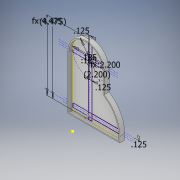
# Autodesk Inventor part: housing
Saved by Autodesk Inventor 2017 (Build 210142000, 142)
## iProperties
Created: 2016-11-23
Part Number: housing
Material: Generic
Document SubType Name: Modeling
Designer: cody
Density: 1 g/cm^3
Appearance: Default
Author: cody
Autodesk Inventor part; units mm, degrees
ref_plane "YZ Plane" through (0, 0, 0) normal (1, 0, 0) x (0, 1, 0)
ref_plane "XZ Plane" through (0, 0, 0) normal (0, 1, 0) x (-1, 0, 0)
ref_plane "XY Plane" through (0, 0, 0) normal (0, 0, 1) x (1, 0, 0)
sketch "Outline" plane through (0, 0, 0) normal (0, 0, 1) x (1, 0, 0)
  line L0 (0, 37.1721) -> (55.88, 37.1721) construction
  line L1 (55.88, 37.1721) -> (55.88, 115.2771) construction
  line L2 (55.88, 115.2771) -> (0, 115.2771) construction
  line L3 (0, 115.2771) -> (0, 37.1721) construction
  circle A0 centre (27.94, 115.2771) radius 26.67 construction
  circle A1 centre (27.94, 37.1721) radius 52.07 construction
  circle A2 centre (27.94, 115.2771) radius 27.94 construction
  circle A3 centre (27.94, 37.1721) radius 53.34 construction
  arc A4 (55.88, 115.2771) -> (0, 115.2771) centre (27.94, 115.2771) ccw
  line L4 (55.88, 115.2771) -> (55.88, 82.609)
  arc A5 (81.28, 37.1721) -> (55.88, 82.609) centre (27.94, 37.1721) ccw
  line L5 (142.2611, 29.5521) -> (-127.7704, 29.5521) construction
  line L6 (81.28, 37.1721) -> (81.28, 29.5521)
  line L7 (0, 29.5521) -> (81.28, 29.5521)
  line L8 (0, 115.2771) -> (0, 29.5521)
  dimension "d20" = 78.105
  dimension "d23" = 104.14
  dimension "d25" = 53.34
  dimension "d27" = 1.27
  dimension "d28" = 55.88
  dimension "d29" = 55.88
  dimension "d30" = 1.27
  dimension "d31" = 7.62
  constraints: 18 end point, 5 centre point, 4 point on circle, 3 horizontal, 3 point on line, 3 vertical, 2 midpoint, 2 parallel, 2 perpendicular, 1 coincident, 1 collinear, 1 tangent, 3 other
  measures "d20" distance of L2.end L0.start
  measures "d23" diameter of A1
  measures "d25" diameter of A0
  measures "d27" radial gap between concentric circles of A0 A2
  measures "d28" diameter of A2
  measures "d29" distance of L1.end L2.end
  measures "d31" distance between parallel lines of L5 L0
extrude "Edge Ext" add sketch "Outline" along normal blind 6.35
shell "Edge_Shell" thickness 1.5875 outward yes removed faces 1 at (18.6267, 75.8128, 6.35)
sketch "Pegs" plane through (27.94, 115.2771, 0) normal (0, 0, 1) x (1, 0, 0)
  arc A0 (53.34, -78.105) -> (27.94, -32.6681) centre (0, -78.105) ccw projected
  circle A1 centre (0, -78.105) radius 1.143
  point P0 (-27.94, -115.2771)
  dimension "d36" = 2.286
  constraints: 1 centre point, 1 coincident
  measures "d36" diameter of A1
extrude "Pegs_Ext" add sketch "Pegs" along normal blind 7.9375
sketch "Sketch3" plane through (27.94, 115.2771, 0) normal (0, 0, 1) x (1, 0, 0)
  circle A0 centre (0, -78.105) radius 1.143 projected
  arc A1 (27.94, 0) -> (-27.94, 0) centre (0, 0) ccw projected
  line L0 (-27.94, 0) -> (-27.94, -85.725) projected
  line L1 (-27.94, -85.725) -> (53.34, -85.725) projected
  line L2 (53.34, -85.725) -> (53.34, -78.105) projected
  arc A2 (53.34, -78.105) -> (27.94, -32.6681) centre (0, -78.105) ccw projected
  line L3 (27.94, -32.6681) -> (27.94, 0) projected
  line L4 (46.559, 0) -> (-50.3798, 0) construction
  line L5 (0, 35.3546) -> (0, -92.7907) construction
  circle A3 centre (0, 0) radius 27.94 construction
  line L6 (46.559, 3.175) -> (-50.3798, 3.175) construction
  line L7 (46.559, -3.175) -> (-50.3798, -3.175) construction
  line L8 (-27.94, 3.175) -> (27.94, 3.175)
  line L9 (27.94, 3.175) -> (27.94, -3.175)
  line L10 (27.94, -3.175) -> (-27.94, -3.175)
  line L11 (-27.94, -3.175) -> (-27.94, 3.175)
  line L12 (3.175, 35.3546) -> (3.175, -85.725) construction
  line L13 (-3.175, 35.3546) -> (-3.175, -92.7907) construction
  line L14 (-3.175, 27.94) -> (3.175, 27.94)
  line L15 (3.175, 27.94) -> (3.175, -85.725)
  line L16 (3.175, -85.725) -> (-3.175, -85.725)
  line L17 (-3.175, -85.725) -> (-3.175, 27.94)
  arc A4 (27.94, 0) -> (-27.94, 0) centre (0, 0) ccw projected
  line L18 (0, -78.105) -> (73.8592, -78.105) construction
  line L19 (0, -78.105) -> (-73.8592, -78.105) construction
  line L20 (71.8226, -74.93) -> (-43.3054, -74.93) construction
  line L21 (71.8226, -81.28) -> (-43.3054, -81.28) construction
  line L22 (-27.94, -74.93) -> (53.34, -74.93)
  line L23 (53.34, -74.93) -> (53.34, -81.28)
  line L24 (53.34, -81.28) -> (-27.94, -81.28)
  line L25 (-27.94, -81.28) -> (-27.94, -74.93)
  arc A5 (53.34, -78.105) -> (27.94, -32.6681) centre (0, -78.105) ccw projected
  line L26 (-27.94, -85.725) -> (-27.94, 0) projected
  point P0 (-27.94, -115.2771)
  dimension "d39" = 3.175
  dimension "d40" = 3.175
  dimension "d41" = 55.88
  dimension "d42" = 55.88
  dimension "d43" = 3.175
  dimension "d44" = 3.175
  dimension "d45" = 113.665
  dimension "d46" = 113.665
  dimension "d47" = 3.175
  constraints: 44 end point, 10 parallel, 7 horizontal, 5 point on line, 3 perpendicular, 3 symmetric about line, 2 tangent, 2 vertical, 1 centre point, 1 coincident, 1 collinear, 1 concentric, 1 other
  measures "d39" distance between parallel lines of L4 L6
  measures "d40" distance between parallel lines of L4 L7
  measures "d41" distance of L8.start L8.end
  measures "d42" diameter of A3
  measures "d43" distance between parallel lines of L5 L12
  measures "d44" distance between parallel lines of L5 L13
  measures "d46" distance between parallel lines of L14 L16
  measures "d47" distance between parallel lines of L20 L18
equation "\"d29\" = d28"
equation "\"d41\" = d42"
equation "\"d46\" = d45"
body "Solid1"
